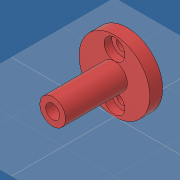
# Autodesk Inventor part: Schalter_Basis_rund
Saved by Autodesk Inventor 2019 (Build 230136000, 136)
## iProperties
Created: 2020-08-07
Part Number: Schalter_Basis_rund
Material: Generisch
Document SubType Name: Modeling
Designer: Stefan
Mass: 3.91933 g
Surface Area: 29.3228 cm^2
Volume: 3.91933 cm^3
Density: 1 g/cm^3
Appearance: Glatt - Rot
Author: Stefan
Autodesk Inventor part; units mm, degrees
ref_plane "YZ Plane" through (0, 0, 0) normal (1, 0, 0) x (0, 1, 0)
ref_plane "XZ Plane" through (0, 0, 0) normal (0, 1, 0) x (-1, 0, 0)
ref_plane "XY Plane" through (0, 0, 0) normal (0, 0, 1) x (1, 0, 0)
sketch "Skizze1" plane through (0, 0, 0) normal (0, 0, 1) x (1, 0, 0)
  circle A0 centre (0, 0) radius 13.75
  circle A1 centre (0, 0) radius 5
  line L0 (0, 13.75) -> (0, -13.75) construction
  circle A2 centre (0, 9) radius 4
  circle A3 centre (0, 9) radius 2.25
  circle A4 centre (0, -9) radius 4
  circle A5 centre (0, -9) radius 2.25
  line L1 (-13.75, 0) -> (13.75, 0) construction
  circle A6 centre (0, 0) radius 2.75
  circle A7 centre (0, 0) radius 3.5
  dimension "d0" = 27.5
  dimension "d1" = 10
  dimension "d4" = 8
  dimension "d5" = 18
  dimension "d6" = 4.5
  dimension "d7" = 5.5
  dimension "d14" = 7
  constraints: 9 coincident, 8 centre point, 5 midpoint, 4 end point, 4 point on circle, 2 equal radius, 2 point on line, 1 horizontal, 1 symmetric about line, 1 vertical
  measures "d0" diameter of A0
  measures "d1" diameter of A1
  measures "d4" diameter of A2
  measures "d5" distance of A4.centre A2.centre
  measures "d6" diameter of A5
  measures "d7" diameter of A6
  measures "d14" diameter of A7
extrude "Extrusion1" add sketch "Skizze1" against normal blind 5 contours A0 | A1 | A4 | A2 | A6 | A7
extrude "Extrusion2" cut sketch "Skizze1" against normal blind 3 contours A4 | A2
extrude "Extrusion3" add sketch "Skizze1" along normal blind 24 contours A1
extrude "Extrusion4" add sketch "Skizze1" along normal blind 24 contours A7
